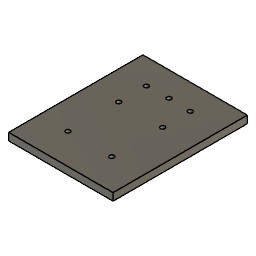
lowChasis (Autodesk Fusion 360 design; units mm, degrees)
part number: 2026-05-16-12-14-17-820
Autodesk Fusion 360 part; units mm, degrees
sketch "Sketch1" plane through (0, 0, 0) normal (0, 1, 0) x (1, 0, 0)
  line L0 (0, 0) -> (-70, 0)
  line L1 (-70, 0) -> (-70, -70)
  line L2 (-70, -70) -> (0, -70)
  line L3 (0, -70) -> (0, 0)
  line L4 (-60, -50) -> (-12, -50) construction
  line L5 (-12, -50) -> (-12, -25) construction
  line L6 (-12, -25) -> (-60, -25) construction
  line L7 (-60, -25) -> (-60, -50) construction
  line L8 (-21.2988, -54.5) -> (-21.2988, -20.5)
  line L9 (-50.7012, -54.5) -> (-50.7012, -20.5)
  line L10 (-60, -37.5) -> (-12, -37.5)
  line L11 (-36, -50) -> (-36, -25)
  line L12 (-21.2988, -54.5) -> (-50.7012, -54.5)
  line L13 (-50.7012, -20.5) -> (-21.2988, -20.5)
  line L14 (0, -70) -> (-70, -70)
  line L15 (-70, -70) -> (-70, -90)
  line L16 (-70, -90) -> (0, -90)
  line L17 (0, -90) -> (0, -70)
  line L18 (-36, -54.5) -> (-36, -73.5)
  line L19 (-50.7012, -54.5) -> (-50.7012, -73)
  line L20 (-21.2988, -54.5) -> (-21.2988, -73)
  point P0 (-21.2988, -54.5)
  point P1 (-50.7012, -54.5)
  point P2 (-50.7012, -20.5)
  point P3 (-21.2988, -20.5)
  point P4 (-36, -54.5)
  point P5 (-36, -54.5)
  point P6 (-50.7012, -54.5)
  point P7 (-36, -54.5)
  point P8 (-21.2988, -54.5)
  point P9 (-50.7012, -20.5)
  point P10 (-21.2988, -20.5)
  dimension "d1" = 70
  dimension "d2" = 70
  dimension "d3" = 48
  dimension "d4" = 25
  dimension "d5" = 34
  dimension "d6" = 34
  dimension "d7" = 19
  constraint vertical L1
  constraint coincident L0.start L3.end
  constraint horizontal L4
  constraint vertical L5
  constraint horizontal L6
  constraint vertical L7
  constraint perpendicular L4 L8
  constraint midpoint L7 L10.start
  constraint midpoint L5 L10.end
  constraint midpoint L4 L11.start
  constraint midpoint L6 L11.end
  constraint perpendicular L9 L12
  constraint symmetric L10 L12 L13
  constraint coincident P8 P0
  constraint coincident P6 P1
  constraint coincident P9 P2
  constraint coincident P3 L8.end
  constraint horizontal L14
  constraint vertical L15
  constraint horizontal L16
  constraint vertical L17
  constraint midpoint L12 P7
  constraint coincident P7 P5
  constraint perpendicular L14 L18
  constraint perpendicular L14 L19
  constraint perpendicular L2 L20
  constraint coincident P10 P3
  measures "d1" distance of L0.start L0.end
  measures "d2" distance of L0.start L2.end
  measures "d3" distance of L4.start L4.end
  measures "d4" distance of L4.start L6.end
  measures "d5" distance of P8 P3
  measures "d6" distance of P6 P9
  measures "d7" distance of P7 L18.end
extrude "Extrude1" add sketch "Sketch1" along normal blind 5
hole "Hole1" at (-50.7012, 0, 73) at (-36, 0, 73.5) at (-21.2988, 0, 73) at (-21.2988, 0, 54.5) at (-50.7012, 0, 54.5) at (-50.7012, 0, 20.5) at (-21.2988, 0, 20.5) direction (0, 1, 0) diameter 3 depth 5 tip angle 180
move_body "Move1" bodies 1 to x (1, 0, 0) y (0, 0, -1) z (0, 1, 0) at (0, 0, 0)
